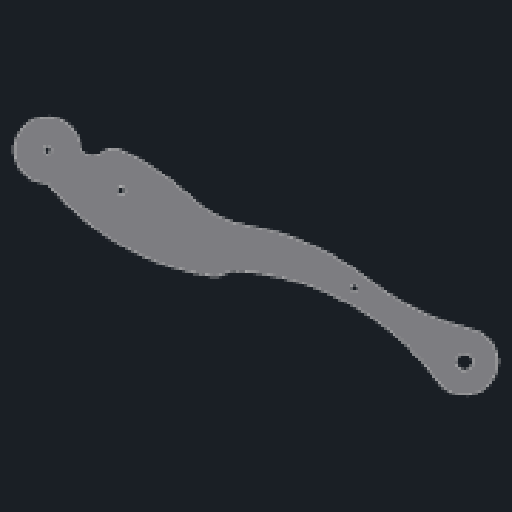
# Autodesk Inventor part: LowerLeg
Saved by Autodesk Inventor 2025.2 (Build 292293000, 293)
## iProperties
Created: 2020-05-17
Part Number: LowerLeg
Material: Generic
Document SubType Name: Sheet Metal
Designer: valer
Density: 1 g/cm^3
Sheet Metal Rule: Default
Appearance: Default
Author: valer
Autodesk Inventor part; units mm, degrees
ref_plane "YZ Plane" through (0, 0, 0) normal (1, 0, 0) x (0, 1, 0)
ref_plane "XZ Plane" through (0, 0, 0) normal (0, 1, 0) x (-1, 0, 0)
ref_plane "XY Plane" through (0, 0, 0) normal (0, 0, 1) x (1, 0, 0)
sketch "Base" plane through (0, 0, 0) normal (0, 0, 1) x (1, 0, 0)
  circle A0 centre (0, 0) radius 25.4
  arc A1 (296.4611, -175.8738) -> (140.4514, -91.7589) centre (131.6761, -294.7694) ccw
  arc A2 (110.2711, -36.5273) -> (55.3611, 0.3584) centre (-26.1088, -180.2356) ccw
  arc A3 (110.2711, -36.5273) -> (151.7939, -57.2356) centre (164.9104, 21.0482) ccw
  arc A4 (244.1, -98.1325) -> (151.7939, -57.2356) centre (118.2154, -257.642) ccw
  arc A5 (244.1, -98.1325) -> (322.9398, -136.302) centre (369.9847, 61.3771) ccw
  arc A6 (339.7063, -172.5127) -> (322.9398, -136.302) centre (317.0592, -161.0119) ccw
  arc A7 (296.4611, -175.8738) -> (339.7063, -172.5127) centre (317.0592, -161.0119) ccw
  line L0 (128.6011, -96.3262) -> (140.4514, -91.7589)
  line L1 (0, 0) -> (317.0592, -161.0119) construction
  circle A8 centre (317.0592, -161.0119) radius 25.4 construction
  arc A9 (0, -25.4) -> (128.6011, -96.3262) centre (153.166, 100.265) ccw
  line L2 (0, 0) -> (0, -25.4) construction
  arc A10 (55.3611, 0.3584) -> (42.3326, -1.2004) centre (50.1387, -11.2181) ccw
  arc A11 (25.4, -0.0141) -> (42.3326, -1.2004) centre (34.5266, 8.8174) ccw
  line L3 (110.2711, -36.5273) -> (102.4101, -52.0068) construction
  line L4 (50.1387, -11.2181) -> (44.3883, -22.5417) construction
  line L5 (140.4514, -91.7589) -> (148.7008, -75.5146) construction
  line L6 (244.1, -98.1325) -> (233.6726, -118.6658) construction
  line L7 (339.7063, -172.5127) -> (317.0592, -161.0119) construction
  dimension "d101" = 50.8
  dimension "d98" = 355.6
  dimension "d99" = 203.2
  dimension "d100" = 79.375
  dimension "d102" = 198.12
  dimension "d103" = 50.8
  dimension "d104" = 12.7
  dimension "d105" = 203.2
  dimension "d106" = 48
  dimension "d107" = 12.7
  dimension "d108" = 12.7
  dimension "d109" = 23.495
  dimension "d111" = 158.75
  dimension "d112" = 222.25
  dimension "d113" = 49.784
  dimension "d114" = 65.0748
  dimension "d115" = 51.9176
  dimension "d116" = 95.3008
  dimension "d117" = 93.5228
  measures "d98" distance of L1.start L1.end
  measures "d99" radius of A4
  measures "d100" radius of A3
  measures "d102" radius of A2
  measures "d103" diameter of A0
  measures "d104" radius of A10
  measures "d105" radius of A5
  measures "d106" angle of L1 L0
  measures "d107" distance of L0.start L0.end
  measures "d108" distance from line of L1 L4.start
  measures "d109" distance from line of L1 A11.centre
  measures "d111" distance from line of L1 A9.centre
  measures "d112" distance from line of L1 A5.centre
  measures "d113" distance from line of point (0, 0) L4
  measures "d114" distance from line of L4.end L3
  measures "d115" distance between parallel lines of L5 L3
  measures "d116" distance between parallel lines of L6 L5
  measures "d117" distance from line of A6.centre L6
extrude "Plate1" add sketch "Base" along normal blind 5.08
sketch "MountHoles" plane through (0, 0, 5.08) normal (0, 0, 1) x (1, 0, 0)
  arc A0 (296.4611, -175.8738) -> (322.9398, -136.302) centre (317.0592, -161.0119) ccw projected
  circle A1 centre (317.0592, -161.0119) radius 3.175
  circle A2 centre (0, 0) radius 3.175
  circle A3 centre (0, 0) radius 15.875 construction
  circle A4 centre (0, 15.875) radius 3.175
  line L0 (0, 15.875) -> (0, 0) construction
  circle A5 centre (-13.7482, 7.9375) radius 3.175
  circle A6 centre (-13.7482, -7.9375) radius 3.175
  circle A7 centre (0, -15.875) radius 3.175
  circle A8 centre (13.7482, -7.9375) radius 3.175
  circle A9 centre (13.7482, 7.9375) radius 3.175
  point P0 (278.6053, -195.7416)
  point P1 (14.9365, 6.9557)
  dimension "d40" = 31.75
  dimension "d38" = 6.35
  dimension "d39" = 6.35
  dimension "d43" = 360
  constraints: 8 centre point, 3 coincident, 2 end point, 1 equal radius, 1 vertical, 1 vertical alignment, 15 other
  measures "d38" diameter of A1
  measures "d39" diameter of A2
hole "MountHolesFeature" at (0, 0, 5.08) direction (0, 0, -1) diameter 6.35 end through all
fillet "SmallFilletsFeature" radius 8 2 edges at (140.4514, -91.7589, 2.54) (128.6011, -96.3262, 2.54)
sketch "WheelMountHole" plane through (0, 0, 5.08) normal (0, 0, 1) x (1, 0, 0)
  arc A0 (296.4611, -175.8738) -> (322.9398, -136.302) centre (317.0592, -161.0119) ccw projected
  circle A1 centre (317.0592, -161.0119) radius 6.35
  point P0 (0, 0)
  point P1 (278.6053, -195.7416)
  dimension "d83" = 12.7
  constraints: 1 centre point, 1 coincident
  measures "d83" diameter of A1
hole "WheelMountHoleFeature" at (317.0592, -161.0119, 5.08) direction (0, 0, -1) diameter 12.7 end through all
sketch "ShockMountHole" plane through (0, 0, 5.08) normal (0, 0, 1) x (1, 0, 0)
  circle A0 centre (56.1234, -30.8576) radius 3.175 projected
  point P0 (0, 0)
hole "ShockMountHoleFeature" at (56.1234, -30.8576, 5.08) direction (0, 0, -1) diameter 6.35 end through all
sketch "Sketch8" plane through (0, 0, 0) normal (0, 0, -1) x (-1, 0, 0)
  circle A0 centre (-233.2261, -105.1103) radius 3
  arc A1 (-151.7939, -57.2356) -> (-244.1, -98.1325) centre (-118.2154, -257.642) ccw projected
  line L0 (-240.9347, -95.6845) -> (-225.5176, -114.5361) construction
  arc A2 (-142.169, -91.8405) -> (-296.4611, -175.8738) centre (-131.6761, -294.7694) ccw projected
  point P0 (0, 0)
  dimension "d120" = 6
  dimension "d121" = 4
  constraints: 2 end point, 2 point on circle, 1 centre point, 1 coincident, 1 midpoint
  measures "d120" diameter of A0
  measures "d121" distance from line of A1.end L0
extrude "Cut1" cut sketch "Sketch8" against normal blind 5.08
equation "\"d66\" = Thickness"
equation "\"d89\" = Thickness"
equation "\"d96\" = Thickness"
equation "\"d37\" = Thickness"
equation "\"BendRadius\" = Thickness"
equation "\"BendReliefWidth\" = Thickness"
equation "\"BendReliefDepth\" = 0.5 * Thickness"
equation "\"CornerReliefSize\" = 4 * Thickness"
equation "\"MinimumRemnant\" = 2 * Thickness"
equation "\"TransitionRadius\" = BendRadius"
equation "\"JacobiRadiusSize\" = BendRadius"
equation "\"GapSize\" = Thickness"
equation "\"Thickness\" = 5.08"
body "Solid1"
